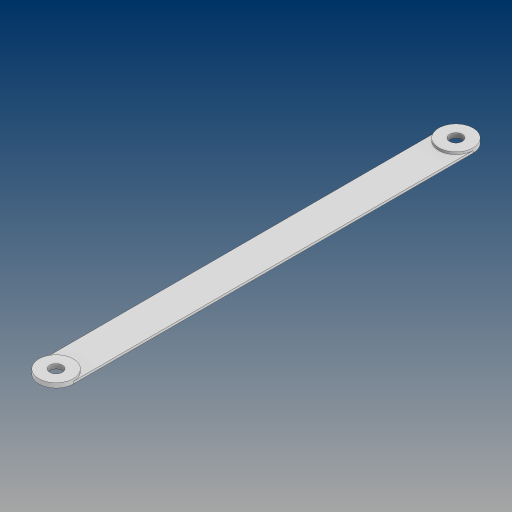
# Autodesk Inventor part: alsoszalagnyomtatasra
Saved by Autodesk Inventor 2023 (Build 270158000, 158)
## iProperties
Created: 2023-11-12
Part Number: alsoszalagnyomtatasra
Material: Generic
Document SubType Name: Modeling
Designer: gd1
Density: 1 g/cm^3
Appearance: Default
Author: gd1
Autodesk Inventor part; units mm, degrees
ref_plane "YZ Plane" through (0, 0, 0) normal (1, 0, 0) x (0, 1, 0)
ref_plane "XZ Plane" through (0, 0, 0) normal (0, 1, 0) x (-1, 0, 0)
ref_plane "XY Plane" through (0, 0, 0) normal (0, 0, 1) x (1, 0, 0)
sketch "Sketch1" plane through (0, 0, 0) normal (0, 1, 0) x (-1, 0, 0)
  circle A0 centre (0, 0) radius 2.75
  line L0 (0, 0) -> (0, -174.842)
  line L1 (0, 0) -> (174.842, 0) construction
  circle A1 centre (0, -174.842) radius 2.75
  line L2 (0, -174.842) -> (0, 0) construction
  line L3 (7.5, -174.842) -> (7.5, 0)
  line L4 (-7.5, 0) -> (-7.5, -174.842)
  arc A2 (-7.5, -174.842) -> (7.5, -174.842) centre (0, -174.842) ccw
  arc A3 (7.5, 0) -> (-7.5, 0) centre (0, 0) ccw
  circle A4 centre (0, 0) radius 7.5
  circle A5 centre (0, -174.842) radius 7.5
  point P0 (0, -87.421)
  dimension "d0" = 5.5
  dimension "d1" = 174.842
  dimension "d2" = 90
  dimension "d3" = 5.5
  dimension "d4" = 15
  constraints: 12 end point, 6 centre point, 6 tangent, 4 coincident, 4 point on circle, 2 vertical, 1 horizontal, 1 midpoint, 1 parallel, 1 perpendicular
  measures "d0" diameter of A0
  measures "d1" distance of L0.start L0.end
  measures "d2" angle of L0 L1
  measures "d3" diameter of A1
  measures "d4" diameter of A3
extrude "Extrusion1" add sketch "Sketch1" along normal blind 2 contours A4 A3 | A5 A2
extrude "Extrusion2" add sketch "Sketch1" along normal blind 1 contours A4 L3 A5 L0 | L0 A5 L4 A4
body "Solid1"
